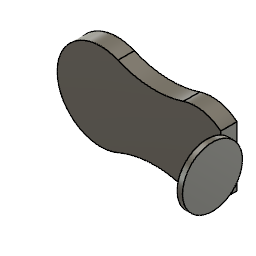
answer (Autodesk Fusion 360 design; units mm, degrees)
part number: 2026-08-05-21-08-28-106
Autodesk Fusion 360 part; units mm, degrees
note: some values were not read from the file. Set by a fixed rule: which sketch regions a step uses.
sketch "Sketch1" plane through (0, 0, 0) normal (1, 0, 0) x (0, 0, -1)
  circle A0 centre (0, 0) radius 27.5
  dimension "d1" = 55
  constraint coincident A0.centre origin
  measures "d1" diameter of A0
extrude "Extrude1" add sketch "Sketch1" along normal blind 5
ref_plane "WorkPlane1" through (0, 0, -27.5) normal (0, 0, 1) x (1, 0, 0)
sketch "Sketch2" plane through (0, 0, -27.5) normal (0, 0, 1) x (1, 0, 0)
  line L0 (0, 0) -> (-150, 0)
  line L1 (0, 0) -> (-23, 0)
  line L2 (-150, 0) -> (-110, 0)
  line L3 (0, 0) -> (0, 27.5)
  circle A0 centre (-23, 0) radius 35.8504
  circle A1 centre (-110, 0) radius 40
  line L4 (0, 27.5) -> (0, -27.5)
  arc A2 (-94.2038, 36.7489) -> (-34.165, 34.0675) centre (-60.6369, 114.8402) ccw
  arc A3 (-34.165, -34.0675) -> (-94.2038, -36.7489) centre (-60.6369, -114.8402) ccw
  point P0 (0, -27.5)
  point P1 (0, 27.5)
  dimension "d6" = 150
  dimension "d7" = 23
  dimension "d8" = 40
  dimension "d9" = 27.5
  dimension "d10" = 85
  constraint coincident L0.start L1.start
  constraint horizontal L0
  constraint parallel L0 L1
  constraint parallel L0 L2
  constraint perpendicular L1 L3
  constraint coincident L1.end A0.centre
  constraint coincident P1 A0
  constraint coincident L0 L2.end
  constraint coincident L0.end A1
  constraint coincident A0 P0
  constraint parallel L3 L4
  constraint coincident A1 A2.start
  constraint coincident A0 A2.end
  constraint tangent A0 A2
  constraint tangent A1 A2
  constraint symmetric L0 A2.end A3.start
  constraint symmetric L0 A2.start A3.end
  constraint symmetric L0 A2 A3
  constraint coincident P0 L4.end
  constraint coincident P1 L3.end
  measures "d6" distance of L0.start L0.end
  measures "d7" distance of L0.start L1.end
  measures "d8" distance of L0.end L2.end
  measures "d9" distance of L0.start L3.end
  measures "d10" radius of A2
extrude "Extrude2" add sketch "Sketch2" along normal blind 15 contours L0 L1 A0 L4 | L0 L1 L3 A0 L4 | L0 A0 A1 A3 | L0 A0 A1 A2 | L0 L2 A1 | L0 L2 A1
